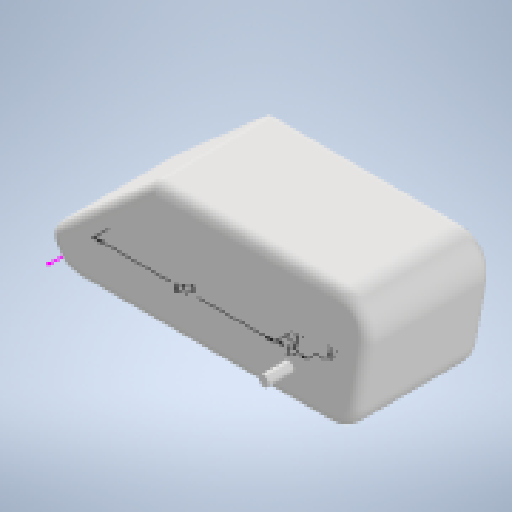
# Autodesk Inventor part: Part6
Saved by Autodesk Inventor 2023 (Build 270158000, 158)
## iProperties
Created: 2023-01-31
Part Number: Part6
Material: Generic
Document SubType Name: Modeling
Designer: oktay
Density: 1 g/cm^3
Appearance: Default
Author: oktay
Autodesk Inventor part; units mm, degrees
ref_plane "YZ Plane" through (0, 0, 0) normal (1, 0, 0) x (0, 1, 0)
ref_plane "XZ Plane" through (0, 0, 0) normal (0, 1, 0) x (-1, 0, 0)
ref_plane "XY Plane" through (0, 0, 0) normal (0, 0, 1) x (1, 0, 0)
sketch "Sketch1" plane through (0, 0, 0) normal (0, 0, 1) x (1, 0, 0)
  line L0 (17.1856, 0) -> (137.4135, 0)
  line L1 (152.1856, 12.3953) -> (157.3147, 41.4837)
  line L2 (0, 0) -> (29.5372, 0) construction
  line L3 (52.5426, 59.0885) -> (142.5426, 59.0885)
  arc A0 (2.1856, 15) -> (17.1856, 0) centre (17.1856, 15) ccw
  arc A1 (157.3147, 41.4837) -> (142.5426, 59.0885) centre (142.5426, 44.0885) ccw
  arc A2 (137.4135, 0) -> (152.1856, 12.3953) centre (137.4135, 15) ccw
  line L4 (2.1856, 15) -> (52.5426, 59.0885)
  point P0 (150, 0)
  point P1 (160.4189, 59.0885)
  point P2 (10.4189, 59.0885)
  dimension "d0" = 150
  dimension "d1" = 60
  dimension "d2" = 100
  dimension "d3" = 60
  dimension "d5" = 15
  dimension "d33" = 150
  dimension "d34" = 90
  constraints: 10 end point, 6 point on circle, 6 point on line, 5 tangent, 3 centre point, 2 equal radius, 2 horizontal
  measures "d0" distance of L2.start point (150, 0)
  measures "d1" distance of point (150, 0) point (160.419, 59.088)
  measures "d2" angle of L1 L0
  measures "d3" distance of L2.start point (10.419, 59.088)
  measures "d5" radius of A0
  measures "d33" horizontal distance of L1.start L4.start
  measures "d34" distance of L3.start L3.end
extrude "Extrusion1" add sketch "Sketch1" along normal blind 40 and the other way blind 20
sketch "Sketch2" plane through (17.1856, 0, 40) normal (0, -1, 0) x (1, 0, 0)
  line L0 (-15, -60) -> (-15, 0) projected
  line L1 (-15, -30) -> (72.5, -30)
  line L2 (72.5, -30) -> (72.5, -27)
  line L3 (72.5, -27) -> (87.5, -27)
  line L4 (87.5, -27) -> (87.5, -33)
  line L5 (87.5, -33) -> (72.5, -33)
  line L6 (72.5, -33) -> (72.5, -30)
  point P0 (-17.1856, -40)
  dimension "d11" = 87.5
  dimension "d12" = 3
  dimension "d13" = 15
  dimension "d14" = 6
  constraints: 12 end point, 5 perpendicular, 1 horizontal, 1 midpoint, 1 point on line
  measures "d11" distance of L1.start L1.end
  measures "d12" distance of L1.end L2.end
  measures "d13" distance of L2.end L3.end
  measures "d14" distance of L3.end L4.end
sketch "Sketch3" plane through (17.1856, 0, 40) normal (0, -1, 0) x (1, 0, 0)
  line L0 (47.5, -33) -> (47.5, -27) projected
  line L1 (47.5, -30) -> (-0.648, -30)
  line L2 (20, -10) -> (30, -10)
  line L3 (45, -25) -> (45, -35)
  line L4 (30, -50) -> (20, -50)
  line L5 (5, -35) -> (5, -25)
  line L6 (5, -10) -> (45, -50) construction
  line L7 (45, -10) -> (5, -50) construction
  arc A0 (20, -10) -> (5, -25) centre (20, -25) ccw
  arc A1 (5, -35) -> (20, -50) centre (20, -35) ccw
  arc A2 (30, -50) -> (45, -35) centre (30, -35) ccw
  arc A3 (45, -25) -> (30, -10) centre (30, -25) ccw
  point P0 (-17.1856, -40)
  point P1 (25, -30)
  dimension "d18" = 40
  dimension "d19" = 40
  dimension "d32" = 15
  constraints: 14 end point, 9 point on line, 8 point on circle, 8 tangent, 4 centre point, 3 equal radius, 3 midpoint, 2 horizontal, 2 parallel, 1 perpendicular
  measures "d18" distance of L6.end L7.end
  measures "d19" distance of L7.start L6.end
  measures "d32" radius of A0
extrude "Extrusion3" cut sketch "Sketch3" against normal blind 10
shell "Shell2" thickness 5 removed faces 5 at (40.519, 3.3333, -10) at (43.8523, 10, 13.3333) at (62.1856, 3.3333, 8.3333) at (22.1856, 3.3333, 11.6667) at (43.8523, 6.6667, 30)
extrude "Extrusion4" cut sketch "Sketch2" against normal blind 26.5
sketch "Sketch4" plane through (62.1856, 0, -10) normal (-1, 0, 0) x (0, 0, 1)
  line L0 (28, 15) -> (12, 15) projected
  line L1 (12, 5) -> (28, 5)
  line L2 (28, 5) -> (28, 15)
  line L3 (28, 15) -> (12, 15)
  line L4 (12, 15) -> (12, 5)
  point P0 (10, 0)
  constraints: 8 end point, 2 parallel, 1 horizontal, 1 perpendicular
extrude "Extrusion5" cut sketch "Sketch4" along normal blind 10 and the other way blind 1.25
sketch "Sketch6" plane through (63.4356, 0, -10) normal (-1, 0, 0) x (0, 0, 1)
  line L0 (-5, 5) -> (45, 5) projected
  line L1 (28.9912, 5) -> (28.9912, 16.326)
  line L2 (28.9912, 16.326) -> (10, 16.326)
  line L3 (10, 16.326) -> (10, 5)
  line L4 (10, 5) -> (14.3032, 5)
  line L5 (28, 5) -> (12, 5) projected
  line L6 (14.3032, 5) -> (14.3032, 11.2314)
  line L7 (14.3032, 11.2314) -> (26.0777, 11.2314)
  line L8 (26.0777, 11.2314) -> (26.0777, 5)
  line L9 (26.0777, 5) -> (28.9912, 5)
  point P0 (10, 0)
  point P1 (26.0777, 5)
  constraints: 16 end point, 4 perpendicular, 4 point on line, 2 vertical, 1 collinear
extrude "Extrusion6" cut sketch "Sketch6" against normal blind 23.25 contours L3 L2 L1 L0 L8 L7 L6
sketch "Sketch7" plane through (63.4356, 0, -10) normal (-1, 0, 0) x (0, 0, 1)
  point P0 (10, 0)
sketch "Sketch8" plane through (17.1856, 0, 40) normal (0, -1, 0) x (1, 0, 0)
  line L0 (72.5, -27) -> (72.5, -33) projected
  line L1 (72.5, -33) -> (87.5, -33) projected
  line L2 (87.5, -27) -> (87.5, -33)
  line L3 (72.5, -33) -> (72.5, -27)
  line L4 (87.5, -27) -> (72.5, -27) projected
  line L5 (72.5, -27) -> (87.5, -27)
  line L6 (87.5, -27) -> (87.5, -25.5)
  line L7 (87.5, -25.5) -> (72.5, -25.5)
  line L8 (72.5, -25.5) -> (72.5, -27)
  line L9 (72.5, -33) -> (87.5, -33)
  line L10 (87.5, -33) -> (87.5, -34.5)
  line L11 (87.5, -34.5) -> (72.5, -34.5)
  line L12 (72.5, -34.5) -> (72.5, -33)
  point P0 (-17.1856, -40)
  dimension "d35" = 15
  dimension "d36" = 1.5
  dimension "d37" = 15
  dimension "d38" = 1.5
  constraints: 20 end point, 5 parallel, 2 horizontal, 2 perpendicular
  measures "d35" distance of L7.end L6.end
  measures "d36" distance of L6.end L5.end
  measures "d37" distance of L10.end L11.end
  measures "d38" distance of L9.end L10.end
extrude "Extrusion7" add sketch "Sketch8" against normal blind 20 contours L8 L7 L6 L4 | L1 L10 L11 L12
sketch "Sketch9" plane through (89.6856, 0, 7) normal (0, 0, 1) x (1, 0, 0)
  line L0 (0, 5) -> (15, 5) projected
  line L1 (0, 5) -> (0, 20) projected
  line L2 (15, 20) -> (0, 20) projected
  line L3 (15, 5) -> (15, 20) projected
  circle A0 centre (7.5, 10) radius 2.5
  point P0 (-89.6856, 0)
  dimension "d41" = 5
  constraints: 1 centre point
  measures "d41" diameter of A0
extrude "Extrusion8" cut sketch "Sketch9" along normal mid plane 37.75 contours A0
fillet "Fillet1" radius 5 16 edges at (154.0333, 53.7303, -20) (154.7502, 26.9395, -20) (147.0553, 3.5093, -20) (77.2996, 0, -20) (6.579, 4.3934, -20) (97.5426, 59.0885, -20) (154.0333, 53.7303, 40) (154.7502, 26.9395, 40) (147.0553, 3.5093, 40) (77.2996, 0, 40) (6.579, 4.3934, 40) (97.5426, 59.0885, 40) (52.5426, 59.0885, 10) (2.1856, 15, 10) (30.9129, 33.5057, -15) (27.3641, 37.0442, 40)
sketch "Sketch12" plane through (0, 0, 40) normal (0, 0, 1) x (1, 0, 0)
  circle A0 centre (118.5745, 15) radius 2.5
  point P0 (0, 0)
  dimension "d51" = 5
  constraints: 1 centre point
  measures "d51" diameter of A0
extrude "Extrusion10" add sketch "Sketch12" along normal blind 12
sketch "Sketch14" plane through (17.1856, 0, -15) normal (0, -1, 0) x (1, 0, 0)
  line L0 (52.9923, 21) -> (58.9923, 21)
  line L1 (58.9923, 21) -> (58.9923, 29)
  line L2 (58.9923, 29) -> (52.9923, 29)
  line L3 (52.9923, 29) -> (52.9923, 21)
  line L4 (72.5, 22) -> (72.5, 28) projected
  point P0 (-17.1856, 15)
  point P1 (72.5, 25)
  point P2 (55.9923, 21)
  dimension "d54" = 6
  dimension "d55" = 8
  dimension "d56" = 4
  constraints: 8 end point, 2 midpoint, 2 parallel, 1 horizontal, 1 perpendicular
  measures "d54" distance of L2.end L1.end
  measures "d55" distance of L1.end L0.end
  measures "d56" vertical distance of point (72.5, 25) point (55.992, 21)
extrude "Extrusion11" cut sketch "Sketch14" against normal blind 10
body "Solid1"
